Autodesk Fusion 360 part; units mm, degrees
(part 11 of 13)
  line L8940 (111.831, -138.081) -> (111.826, -138.08)
  line L8941 (112.571, -138.625) -> (112.501, -138.633)
  line L8942 (112.241, -138.364) -> (112.216, -138.337)
  line L8943 (111.159, -137.961) -> (111.159, -137.961)
  line L8944 (111.608, -138.003) -> (111.39, -137.964)
  line L8945 (113.035, -138.178) -> (112.933, -138.254)
  line L8946 (112.854, -138.314) -> (112.694, -138.481)
  line L8947 (110.495, -138.178) -> (110.393, -138.254)
  line L8948 (109.961, -138.633) -> (109.897, -138.602)
  line L8949 (111.39, -137.964) -> (111.385, -137.964)
  line L8950 (110.031, -138.625) -> (109.961, -138.633)
  line L8951 (112.626, -138.58) -> (112.571, -138.625)
  line L8952 (112.933, -138.254) -> (112.854, -138.314)
  line L8953 (109.835, -138.513) -> (109.832, -138.508)
  line L8954 (111.312, -137.963) -> (111.159, -137.961)
  line L8955 (112.375, -138.513) -> (112.372, -138.508)
  line L8956 (109.897, -138.602) -> (109.876, -138.577)
  line L8957 (109.812, -138.487) -> (109.701, -138.364)
  line L8958 (112.034, -138.193) -> (112.03, -138.191)
  line L8959 (111.618, -138.006) -> (111.618, -138.006)
  line L8960 (103.048, -123.079) -> (103.053, -123.008)
  line L8961 (103.139, -122.872) -> (103.132, -122.822)
  line L8962 (109.343, -129.567) -> (109.34, -129.559)
  line L8963 (103.096, -122.951) -> (103.146, -122.933)
  line L8964 (109.328, -129.501) -> (109.314, -129.467)
  line L8965 (109.411, -138.147) -> (109.361, -138.097)
  line L8966 (103.144, -117.596) -> (103.151, -117.577)
  line L8967 (109.202, -129.261) -> (109.189, -129.246)
  line L8968 (109.343, -129.575) -> (109.343, -129.567)
  line L8969 (109.346, -129.746) -> (109.346, -129.735)
  line L8970 (102.915, -121.335) -> (103.012, -121.185)
  line L8971 (109.498, -138.197) -> (109.494, -138.193)
  line L8972 (109.346, -129.659) -> (109.346, -129.655)
  line L8973 (103.132, -122.822) -> (103.132, -122.314)
  line L8974 (109.239, -129.314) -> (109.221, -129.282)
  line L8975 (102.906, -122.026) -> (102.849, -121.857)
  line L8976 (109.182, -129.236) -> (109.177, -129.23)
  line L8977 (103.132, -117.697) -> (103.14, -117.647)
  line L8978 (109.348, -129.727) -> (109.346, -129.659)
  line L8979 (103.122, -122.307) -> (102.998, -122.179)
  line L8980 (102.998, -122.179) -> (102.906, -122.026)
  line L8981 (109.344, -129.611) -> (109.343, -129.575)
  line L8982 (109.314, -129.467) -> (109.31, -129.456)
  line L8983 (109.31, -129.456) -> (109.3, -129.421)
  line L8984 (109.328, -129.501) -> (109.328, -129.501)
  line L8985 (109.346, -138.037) -> (109.346, -129.746)
  line L8986 (109.345, -129.623) -> (109.344, -129.611)
  line L8987 (109.298, -129.413) -> (109.288, -129.396)
  line L8988 (109.279, -129.378) -> (109.272, -129.359)
  line L8989 (109.346, -129.655) -> (109.346, -129.627)
  line L8990 (109.337, -129.548) -> (109.333, -129.528)
  line L8991 (109.331, -129.516) -> (109.33, -129.508)
  line L8992 (109.272, -129.359) -> (109.246, -129.324)
  line L8993 (109.288, -129.396) -> (109.279, -129.378)
  line L8994 (109.3, -129.421) -> (109.298, -129.413)
  line L8995 (109.246, -129.324) -> (109.239, -129.314)
  line L8996 (110.7, -138.07) -> (110.7, -138.07)
  line L8997 (109.361, -138.097) -> (109.346, -138.037)
  line L8998 (109.876, -138.577) -> (109.835, -138.513)
  line L8999 (109.346, -129.627) -> (109.345, -129.623)
  line L9000 (109.494, -138.193) -> (109.411, -138.147)
  line L9001 (109.34, -129.559) -> (109.337, -129.548)
  line L9002 (109.34, -129.559) -> (109.34, -129.559)
  line L9003 (109.333, -129.528) -> (109.331, -129.516)
  line L9004 (103.012, -121.185) -> (103.132, -121.068)
  line L9005 (109.33, -129.508) -> (109.328, -129.501)
  line L9006 (103.142, -122.923) -> (103.139, -122.872)
  line L9007 (109.346, -129.735) -> (109.348, -129.727)
  line L9008 (104.249, -109.045) -> (104.184, -109.088)
  line L9009 (109.135, -129.194) -> (103.082, -123.141)
  line L9010 (109.177, -129.23) -> (109.143, -129.202)
  line L9011 (96.4732, -108.552) -> (94.3232, -108.552)
  line L9012 (103.146, -122.933) -> (103.142, -122.923)
  line L9013 (94.3232, -108.552) -> (94.3232, -113.452)
  line L9014 (84.9232, -102.652) -> (94.3232, -102.652)
  line L9015 (103.151, -117.577) -> (103.154, -117.557)
  line L9016 (104.088, -109.107) -> (102.838, -109.107)
  line L9017 (94.3232, -102.652) -> (94.3232, -107.552)
  line L9018 (84.9232, -113.452) -> (84.9232, -102.652)
  line L9019 (102.588, -108.552) -> (101.073, -108.552)
  line L9020 (102.661, -109.034) -> (102.607, -108.953)
  line L9021 (101.073, -108.602) -> (96.4732, -108.602)
  line L9022 (96.4732, -108.602) -> (96.4732, -108.552)
  line L9023 (102.607, -108.953) -> (102.588, -108.857)
  line L9024 (103.082, -123.141) -> (103.048, -123.079)
  line L9025 (109.143, -129.202) -> (109.135, -129.194)
  line L9026 (103.154, -117.557) -> (103.176, -117.511)
  line L9027 (103.132, -121.068) -> (103.132, -117.704)
  line L9028 (109.189, -129.246) -> (109.182, -129.236)
  line L9029 (103.132, -117.704) -> (103.132, -117.697)
  line L9030 (109.221, -129.282) -> (109.221, -129.282)
  line L9031 (103.132, -122.314) -> (103.122, -122.307)
  line L9032 (103.193, -117.463) -> (103.206, -117.447)
  line L9033 (99.2801, -138.842) -> (99.3742, -139.005)
  line L9034 (102.832, -121.679) -> (102.854, -121.502)
  line L9035 (109.221, -129.282) -> (109.217, -129.276)
  line L9036 (109.217, -129.276) -> (109.202, -129.261)
  line L9037 (103.214, -117.429) -> (103.248, -117.391)
  line L9038 (102.742, -109.088) -> (102.661, -109.034)
  line L9039 (103.14, -117.647) -> (103.144, -117.596)
  line L9040 (103.206, -117.447) -> (103.214, -117.429)
  line L9041 (102.849, -121.857) -> (102.832, -121.679)
  line L9042 (103.053, -123.008) -> (103.096, -122.951)
  line L9043 (104.184, -109.088) -> (104.088, -109.107)
  line L9044 (99.1542, -138.702) -> (99.2801, -138.842)
  line L9045 (104.96, -109.045) -> (104.249, -109.045)
  line L9046 (102.838, -109.107) -> (102.742, -109.088)
  line L9047 (105.951, -114.677) -> (105.951, -110.037)
  line L9048 (103.176, -117.511) -> (103.193, -117.463)
  line L9049 (103.248, -117.391) -> (103.278, -117.35)
  line L9050 (102.854, -121.502) -> (102.915, -121.335)
  line L9051 (103.278, -117.35) -> (105.951, -114.677)
  line L9052 (98.8301, -138.515) -> (99.002, -138.591)
  line L9053 (105.951, -110.037) -> (104.96, -109.045)
  line L9054 (102.588, -108.857) -> (102.588, -108.552)
  line L9055 (101.073, -108.552) -> (101.073, -108.602)
  line L9056 (113.064, -138.842) -> (113.19, -138.702)
  line L9057 (111.854, -138.702) -> (111.98, -138.842)
  line L9058 (113.886, -140.266) -> (113.698, -140.266)
  line L9059 (112.97, -139.005) -> (113.064, -138.842)
  line L9060 (114.242, -140.15) -> (114.07, -140.227)
  line L9061 (97.8239, -139.9) -> (97.7298, -139.737)
  line L9062 (98.6461, -140.266) -> (98.4579, -140.266)
  line L9063 (99.002, -138.591) -> (99.1542, -138.702)
  line L9064 (114.394, -138.702) -> (114.52, -138.842)
  line L9065 (98.2739, -140.227) -> (98.102, -140.15)
  line L9066 (114.242, -138.591) -> (114.394, -138.702)
  line L9067 (111.98, -138.842) -> (112.074, -139.005)
  line L9068 (98.2739, -138.515) -> (98.4579, -138.476)
  line L9069 (97.6717, -139.558) -> (97.652, -139.371)
  line L9070 (114.672, -139.183) -> (114.692, -139.371)
  line L9071 (114.614, -139.737) -> (114.52, -139.9)
  line L9072 (97.7298, -139.005) -> (97.8239, -138.842)
  line L9073 (114.614, -139.005) -> (114.672, -139.183)
  line L9074 (98.4579, -138.476) -> (98.6461, -138.476)
  line L9075 (98.102, -138.591) -> (98.2739, -138.515)
  line L9076 (113.514, -138.515) -> (113.698, -138.476)
  line L9077 (97.9498, -138.702) -> (98.102, -138.591)
  line L9078 (114.07, -138.515) -> (114.242, -138.591)
  line L9079 (99.2801, -139.9) -> (99.1542, -140.039)
  line L9080 (97.7298, -139.737) -> (97.6717, -139.558)
  line L9081 (98.8301, -140.227) -> (98.6461, -140.266)
  line L9082 (114.52, -138.842) -> (114.614, -139.005)
  line L9083 (99.452, -139.371) -> (99.4323, -139.558)
  line L9084 (97.8239, -138.842) -> (97.9498, -138.702)
  line L9085 (112.97, -139.737) -> (112.912, -139.558)
  line L9086 (94.3232, -113.452) -> (84.9232, -113.452)
  line L9087 (113.342, -140.15) -> (113.19, -140.039)
  line L9088 (112.132, -139.558) -> (112.074, -139.737)
  line L9089 (97.6717, -139.183) -> (97.7298, -139.005)
  line L9090 (114.692, -139.371) -> (114.672, -139.558)
  line L9091 (113.064, -139.9) -> (112.97, -139.737)
  line L9092 (97.9498, -140.039) -> (97.8239, -139.9)
  line L9093 (99.1542, -140.039) -> (99.002, -140.15)
  line L9094 (99.3742, -139.737) -> (99.2801, -139.9)
  line L9095 (99.4323, -139.183) -> (99.452, -139.371)
  line L9096 (99.4323, -139.558) -> (99.3742, -139.737)
  line L9097 (99.002, -140.15) -> (98.8301, -140.227)
  line L9098 (112.912, -139.183) -> (112.97, -139.005)
  line L9099 (98.4579, -140.266) -> (98.2739, -140.227)
  line L9100 (98.102, -140.15) -> (97.9498, -140.039)
  line L9101 (99.3742, -139.005) -> (99.4323, -139.183)
  line L9102 (98.6461, -138.476) -> (98.8301, -138.515)
  line L9103 (97.652, -139.371) -> (97.6717, -139.183)
  line L9104 (110.802, -138.591) -> (110.974, -138.515)
  line L9105 (114.07, -140.227) -> (113.886, -140.266)
  line L9106 (112.132, -139.183) -> (112.152, -139.371)
  line L9107 (113.19, -138.702) -> (113.342, -138.591)
  line L9108 (113.698, -138.476) -> (113.886, -138.476)
  line L9109 (111.53, -138.515) -> (111.702, -138.591)
  line L9110 (112.074, -139.005) -> (112.132, -139.183)
  line L9111 (102.994, -115.901) -> (103.105, -115.958)
  line L9112 (110.372, -139.183) -> (110.43, -139.005)
  line L9113 (110.43, -139.737) -> (110.372, -139.558)
  line L9114 (103.105, -116.605) -> (102.994, -116.662)
  line L9115 (111.346, -138.476) -> (111.53, -138.515)
  line L9116 (111.702, -140.15) -> (111.53, -140.227)
  line L9117 (103.25, -116.158) -> (103.27, -116.281)
  line L9118 (103.27, -116.281) -> (103.25, -116.405)
  line L9119 (103.25, -116.405) -> (103.194, -116.516)
  line L9120 (110.802, -140.15) -> (110.65, -140.039)
  line L9121 (111.702, -138.591) -> (111.854, -138.702)
  line L9122 (110.43, -139.005) -> (110.524, -138.842)
  line L9123 (112.074, -139.737) -> (111.98, -139.9)
  line L9124 (102.87, -116.681) -> (102.746, -116.662)
  line L9125 (112.152, -139.371) -> (112.132, -139.558)
  line L9126 (113.342, -138.591) -> (113.514, -138.515)
  line L9127 (114.672, -139.558) -> (114.614, -139.737)
  line L9128 (103.105, -115.958) -> (103.194, -116.046)
  line L9129 (103.194, -116.046) -> (103.25, -116.158)
  line L9130 (103.194, -116.516) -> (103.105, -116.605)
  line L9131 (111.854, -140.039) -> (111.702, -140.15)
  line L9132 (111.158, -140.266) -> (110.974, -140.227)
  line L9133 (111.98, -139.9) -> (111.854, -140.039)
  line L9134 (110.524, -139.9) -> (110.43, -139.737)
  line L9135 (112.892, -139.371) -> (112.912, -139.183)
  line L9136 (114.52, -139.9) -> (114.394, -140.039)
  line L9137 (113.19, -140.039) -> (113.064, -139.9)
  line L9138 (102.994, -116.662) -> (102.87, -116.681)
  line L9139 (110.352, -139.371) -> (110.372, -139.183)
  line L9140 (110.974, -138.515) -> (111.158, -138.476)
  line L9141 (113.886, -138.476) -> (114.07, -138.515)
  line L9142 (113.514, -140.227) -> (113.342, -140.15)
  line L9143 (110.524, -138.842) -> (110.65, -138.702)
  line L9144 (112.912, -139.558) -> (112.892, -139.371)
  line L9145 (111.53, -140.227) -> (111.346, -140.266)
  line L9146 (113.698, -140.266) -> (113.514, -140.227)
  line L9147 (110.65, -138.702) -> (110.802, -138.591)
  line L9148 (110.372, -139.558) -> (110.352, -139.371)
  line L9149 (110.65, -140.039) -> (110.524, -139.9)
  line L9150 (114.394, -140.039) -> (114.242, -140.15)
  line L9151 (111.346, -140.266) -> (111.158, -140.266)
  line L9152 (102.553, -123.685) -> (102.129, -123.26)
  line L9153 (102.342, -123.12) -> (102.73, -123.508)
  line L9154 (108.818, -129.602) -> (108.822, -129.607)
  line L9155 (108.837, -129.667) -> (108.837, -138.482)
  line L9156 (107.984, -139.9) -> (107.89, -139.737)
  line L9157 (102.73, -123.508) -> (108.8, -129.579)
  line L9158 (109.162, -140.15) -> (108.99, -140.227)
  line L9159 (109.44, -139.9) -> (109.314, -140.039)
  line L9160 (102.517, -116.458) -> (102.49, -116.405)
  line L9161 (102.693, -116.635) -> (102.342, -116.986)
  line L9162 (111.158, -138.476) -> (111.346, -138.476)
  line L9163 (109.592, -139.183) -> (109.612, -139.371)
  line L9164 (108.262, -140.15) -> (108.11, -140.039)
  line L9165 (108.8, -129.579) -> (108.814, -129.596)
  line L9166 (102.097, -116.899) -> (102.114, -116.873)
  line L9167 (102.47, -116.281) -> (102.49, -116.158)
  line L9168 (108.99, -138.515) -> (109.162, -138.591)
  line L9169 (108.618, -140.266) -> (108.434, -140.227)
  line L9170 (108.99, -140.227) -> (108.806, -140.266)
  line L9171 (110.974, -140.227) -> (110.802, -140.15)
  line L9172 (109.314, -138.702) -> (109.44, -138.842)
  line L9173 (108.828, -129.637) -> (108.837, -129.667)
  line L9174 (109.162, -138.591) -> (109.314, -138.702)
  line L9175 (108.434, -138.515) -> (108.587, -138.482)
  line L9176 (102.73, -123.508) -> (102.73, -123.508)
  line L9177 (107.812, -139.371) -> (107.832, -139.183)
  line L9178 (109.612, -139.371) -> (109.592, -139.558)
  line L9179 (108.434, -140.227) -> (108.262, -140.15)
  line L9180 (108.837, -138.482) -> (108.99, -138.515)
  line L9181 (109.44, -138.842) -> (109.534, -139.005)
  line L9182 (102.49, -116.405) -> (102.47, -116.281)
  line L9183 (108.11, -138.702) -> (108.262, -138.591)
  line L9184 (109.592, -139.558) -> (109.534, -139.737)
  line L9185 (109.534, -139.737) -> (109.44, -139.9)
  line L9186 (102.342, -116.986) -> (102.342, -123.12)
  line L9187 (102.129, -123.26) -> (102.115, -123.243)
  line L9188 (108.262, -138.591) -> (108.434, -138.515)
  line L9189 (108.817, -129.599) -> (108.818, -129.602)
  line L9190 (109.534, -139.005) -> (109.592, -139.183)
  line L9191 (102.111, -123.237) -> (102.107, -123.232)
  line L9192 (108.822, -129.607) -> (108.828, -129.637)
  line L9193 (109.314, -140.039) -> (109.162, -140.15)
  line L9194 (108.814, -129.596) -> (108.817, -129.599)
  line L9195 (102.553, -123.685) -> (102.553, -123.685)
  line L9196 (102.746, -116.662) -> (102.693, -116.635)
  line L9197 (102.107, -123.232) -> (102.101, -123.202)
  line L9198 (108.806, -140.266) -> (108.618, -140.266)
  line L9199 (108.11, -140.039) -> (107.984, -139.9)
  line L9200 (105.894, -138.515) -> (106.078, -138.476)
  line L9201 (106.622, -140.15) -> (106.45, -140.227)
  line L9202 (106.994, -139.737) -> (106.9, -139.9)
  line L9203 (102.87, -115.881) -> (102.994, -115.901)
  line L9204 (105.444, -138.842) -> (105.57, -138.702)
  line L9205 (102.092, -116.934) -> (102.095, -116.912)
  line L9206 (106.622, -138.591) -> (106.774, -138.702)
  line L9207 (105.57, -138.702) -> (105.722, -138.591)
  line L9208 (105.722, -138.591) -> (105.894, -138.515)
  line L9209 (102.115, -123.243) -> (102.112, -123.24)
  line L9210 (102.546, -116.046) -> (102.635, -115.958)
  line L9211 (102.746, -115.901) -> (102.87, -115.881)
  line L9212 (107.832, -139.183) -> (107.89, -139.005)
  line L9213 (106.774, -138.702) -> (106.9, -138.842)
  line L9214 (102.114, -116.873) -> (102.129, -116.846)
  line L9215 (108.587, -138.482) -> (108.587, -129.719)
  line L9216 (105.292, -139.183) -> (105.35, -139.005)
  line L9217 (107.89, -139.005) -> (107.984, -138.842)
  line L9218 (102.129, -116.846) -> (102.517, -116.458)
  line L9219 (102.095, -116.912) -> (102.095, -116.908)
  line L9220 (106.994, -139.005) -> (107.052, -139.183)
  line L9221 (105.292, -139.558) -> (105.272, -139.371)
  line L9222 (105.57, -140.039) -> (105.444, -139.9)
  line L9223 (102.112, -123.24) -> (102.111, -123.237)
  line L9224 (102.095, -116.908) -> (102.096, -116.905)
  line L9225 (107.984, -138.842) -> (108.11, -138.702)
  line L9226 (106.774, -140.039) -> (106.622, -140.15)
  line L9227 (107.072, -139.371) -> (107.052, -139.558)
  line L9228 (105.722, -140.15) -> (105.57, -140.039)
  line L9229 (107.052, -139.558) -> (106.994, -139.737)
  line L9230 (102.635, -115.958) -> (102.746, -115.901)
  line L9231 (105.894, -140.227) -> (105.722, -140.15)
  line L9232 (105.35, -139.737) -> (105.292, -139.558)
  line L9233 (107.052, -139.183) -> (107.072, -139.371)
  line L9234 (105.444, -139.9) -> (105.35, -139.737)
  line L9235 (106.45, -138.515) -> (106.622, -138.591)
  line L9236 (102.101, -123.202) -> (102.092, -123.172)
  line L9237 (107.89, -139.737) -> (107.832, -139.558)
  line L9238 (106.45, -140.227) -> (106.266, -140.266)
  line L9239 (108.587, -129.719) -> (102.553, -123.685)
  line L9240 (102.49, -116.158) -> (102.546, -116.046)
  line L9241 (107.832, -139.558) -> (107.812, -139.371)
  line L9242 (106.078, -140.266) -> (105.894, -140.227)
  line L9243 (105.272, -139.371) -> (105.292, -139.183)
  line L9244 (102.092, -123.172) -> (102.092, -116.934)
  line L9245 (102.096, -116.905) -> (102.097, -116.899)
  line L9246 (106.9, -138.842) -> (106.994, -139.005)
  line L9247 (105.35, -139.005) -> (105.444, -138.842)
  line L9248 (100.248, -122.697) -> (100.252, -122.7)
  line L9249 (100.864, -122.984) -> (101.092, -123.004)
  line L9250 (99.891, -122.256) -> (99.9362, -122.308)
  line L9251 (101.585, -123.228) -> (101.586, -123.272)
  line L9252 (101.635, -123.432) -> (101.641, -123.443)
  line L9253 (101.596, -123.311) -> (101.599, -123.331)
  line L9254 (101.641, -123.443) -> (101.65, -123.461)
  line L9255 (101.496, -122.958) -> (101.555, -122.998)
  line L9256 (101.092, -123.004) -> (101.32, -122.984)
  line L9257 (106.266, -140.266) -> (106.078, -140.266)
  line L9258 (100.44, -122.83) -> (100.44, -122.83)
  line L9259 (99.9522, -122.342) -> (99.9545, -122.347)
  line L9260 (101.555, -122.998) -> (101.583, -123.063)
  line L9261 (106.9, -139.9) -> (106.774, -140.039)
  line L9262 (100.6, -122.905) -> (100.643, -122.925)
  line L9263 (101.584, -123.093) -> (101.583, -123.104)
  line L9264 (106.266, -138.476) -> (106.45, -138.515)
  line L9265 (99.9576, -122.352) -> (100.074, -122.518)
  line L9266 (100.648, -122.926) -> (100.648, -122.926)
  line L9267 (100.643, -122.925) -> (100.648, -122.926)
  line L9268 (101.425, -122.956) -> (101.496, -122.958)
  line L9269 (101.583, -123.063) -> (101.584, -123.078)
  line L9270 (100.252, -122.7) -> (100.252, -122.7)
  line L9271 (100.435, -122.828) -> (100.44, -122.83)
  line L9272 (101.619, -123.383) -> (101.631, -123.426)
  line L9273 (101.584, -123.078) -> (101.584, -123.093)
  line L9274 (99.9522, -122.342) -> (99.9522, -122.342)
  line L9275 (101.584, -123.184) -> (101.584, -123.212)
  line L9276 (101.581, -123.112) -> (101.582, -123.12)
  line L9277 (101.601, -123.338) -> (101.601, -123.338)
  line L9278 (101.635, -123.432) -> (101.635, -123.432)
  line L9279 (101.586, -123.272) -> (101.592, -123.291)
  line L9280 (100.31, -122.741) -> (100.435, -122.828)
  line L9281 (99.9362, -122.308) -> (99.9522, -122.342)
  line L9282 (100.074, -122.518) -> (100.086, -122.535)
  line L9283 (99.9545, -122.347) -> (99.9576, -122.352)
  line L9284 (100.859, -122.983) -> (100.859, -122.983)
  line L9285 (106.078, -138.476) -> (106.266, -138.476)
  line L9286 (100.859, -122.983) -> (100.864, -122.984)
  line L9287 (100.44, -122.83) -> (100.6, -122.905)
  line L9288 (101.32, -122.984) -> (101.425, -122.956)
  line L9289 (100.252, -122.7) -> (100.31, -122.741)
  line L9290 (100.648, -122.926) -> (100.859, -122.983)
  line L9291 (101.631, -123.426) -> (101.635, -123.432)
  line L9292 (101.583, -123.104) -> (101.581, -123.112)
  line L9293 (101.584, -123.216) -> (101.584, -123.216)
  line L9294 (101.657, -123.48) -> (101.662, -123.486)
  line L9295 (100.086, -122.535) -> (100.248, -122.697)
  line L9296 (102.137, -123.988) -> (108.042, -129.892)
  line L9297 (107.295, -138.513) -> (107.292, -138.508)
  line L9298 (107.614, -138.481) -> (107.546, -138.58)
  line L9299 (107.546, -138.58) -> (107.491, -138.625)
  line L9300 (101.601, -123.338) -> (101.615, -123.372)
  line L9301 (101.74, -123.593) -> (101.752, -123.609)
  line L9302 (108.058, -138.104) -> (108.011, -138.148)
  line L9303 (101.712, -123.563) -> (101.727, -123.578)
  line L9304 (107.357, -138.602) -> (107.336, -138.577)
  line L9305 (101.583, -123.18) -> (101.584, -123.184)
  line L9306 (107.959, -138.175) -> (107.955, -138.178)
  line L9307 (101.599, -123.331) -> (101.601, -123.338)
  line L9308 (101.615, -123.372) -> (101.619, -123.383)
  line L9309 (101.584, -123.216) -> (101.584, -123.216)
  line L9310 (101.683, -123.515) -> (101.69, -123.525)
  line L9311 (101.662, -123.486) -> (101.683, -123.515)
  line L9312 (107.963, -138.172) -> (107.959, -138.175)
  line L9313 (108.011, -138.148) -> (107.963, -138.172)
  line L9314 (108.078, -138.036) -> (108.058, -138.104)
  line L9315 (107.272, -138.487) -> (107.161, -138.364)
  line L9316 (108.076, -129.955) -> (108.078, -129.982)
  line L9317 (101.758, -123.614) -> (101.786, -123.637)
  line L9318 (107.491, -138.625) -> (107.421, -138.633)
  line L9319 (101.65, -123.461) -> (101.657, -123.48)
  line L9320 (107.877, -138.236) -> (107.774, -138.314)
  line L9321 (107.292, -138.508) -> (107.272, -138.487)
  line L9322 (107.774, -138.314) -> (107.614, -138.481)
  line L9323 (101.69, -123.525) -> (101.712, -123.563)
  line L9324 (101.584, -123.216) -> (101.585, -123.228)
  line L9325 (101.786, -123.637) -> (101.794, -123.645)
  line L9326 (101.582, -123.12) -> (101.583, -123.18)
  line L9327 (101.584, -123.212) -> (101.584, -123.216)
  line L9328 (101.592, -123.291) -> (101.596, -123.311)
  line L9329 (101.794, -123.645) -> (102.137, -123.988)
  line L9330 (107.421, -138.633) -> (107.357, -138.602)
  line L9331 (101.727, -123.578) -> (101.74, -123.593)
  line L9332 (101.662, -123.486) -> (101.662, -123.486)
  line L9333 (101.582, -123.12) -> (101.582, -123.12)
  line L9334 (107.955, -138.178) -> (107.955, -138.178)
  line L9335 (143.647, -107.958) -> (143.617, -107.965)
  line L9336 (146.657, -97.0052) -> (146.58, -97.0204)
  line L9337 (146.58, -97.0204) -> (146.18, -97.0204)
  line L9338 (145.842, -97.9436) -> (145.841, -97.9461)
  line L9339 (145.98, -96.8204) -> (145.98, -96.6704)
  line L9340 (144.928, -106.657) -> (144.926, -106.66)
  line L9341 (141.756, -124.03) -> (143.626, -122.159)
  line L9342 (144.925, -106.666) -> (144.909, -106.692)
  line L9343 (143.102, -107.973) -> (142.568, -108.508)
  line L9344 (146.104, -97.0052) -> (146.039, -96.9618)
  line L9345 (145.98, -96.6704) -> (145.845, -96.6704)
  line L9346 (145.995, -96.8969) -> (145.98, -96.8204)
  line L9347 (145.845, -96.6704) -> (145.845, -97.917)
  line L9348 (146.104, -96.0856) -> (146.18, -96.0704)
  line L9349 (146.722, -96.9618) -> (146.657, -97.0052)
  line L9350 (146.18, -97.0204) -> (146.104, -97.0052)
  line L9351 (122.753, -122.378) -> (122.752, -122.381)
  line L9352 (122.734, -122.413) -> (122.72, -122.44)
  line L9353 (143.658, -107.95) -> (143.655, -107.954)
  line L9354 (107.185, -117.298) -> (107.296, -117.355)
  line L9355 (143.588, -107.973) -> (143.102, -107.973)
  line L9356 (107.689, -118.134) -> (107.692, -118.137)
  line L9357 (146.765, -96.1939) -> (146.78, -96.2704)
  line L9358 (145.841, -97.9461) -> (145.84, -97.9525)
  line L9359 (146.765, -96.8969) -> (146.722, -96.9618)
  line L9360 (143.655, -107.954) -> (143.653, -107.954)
  line L9361 (145.845, -97.917) -> (145.842, -97.939)
  line L9362 (144.93, -98.8832) -> (144.93, -106.631)
  line L9363 (146.039, -96.9618) -> (145.995, -96.8969)
  line L9364 (144.93, -106.631) -> (144.927, -106.653)
  line L9365 (145.842, -97.939) -> (145.842, -97.9436)
  line L9366 (143.617, -107.965) -> (143.588, -107.973)
  line L9367 (144.927, -106.653) -> (144.928, -106.657)
  line L9368 (145.823, -97.9784) -> (145.808, -98.0054)
  line L9369 (107.675, -118.116) -> (107.689, -118.134)
  line L9370 (107.693, -118.139) -> (107.697, -118.145)
  line L9371 (145.84, -97.9525) -> (145.823, -97.9784)
  line L9372 (144.894, -106.719) -> (143.676, -107.937)
  line L9373 (145.808, -98.0054) -> (144.93, -98.8832)
  line L9374 (146.78, -96.2704) -> (146.78, -96.8204)
  line L9375 (107.692, -118.137) -> (107.693, -118.139)
  line L9376 (146.58, -96.0704) -> (146.657, -96.0856)
  line L9377 (144.909, -106.692) -> (144.894, -106.719)
  line L9378 (143.676, -107.937) -> (143.658, -107.95)
  line L9379 (108.038, -123.102) -> (108.967, -124.03)
  line L9380 (144.926, -106.66) -> (144.925, -106.666)
  line L9381 (146.657, -96.0856) -> (146.722, -96.129)
  line L9382 (143.653, -107.954) -> (143.647, -107.958)
  line L9383 (122.756, -122.352) -> (122.753, -122.374)
  line L9384 (142.546, -112.787) -> (142.532, -112.814)
  line L9385 (133.148, -113.968) -> (130.702, -116.413)
  line L9386 (130.614, -116.45) -> (123.809, -116.45)
  line L9387 (122.753, -122.374) -> (122.753, -122.378)
  line L9388 (141.414, -113.931) -> (141.396, -113.945)
  line L9389 (121.924, -123.205) -> (121.895, -123.213)
  line L9390 (114.261, -122.337) -> (114.122, -122.419)
  line L9391 (113.953, -122.474) -> (113.775, -122.49)
  line L9392 (115.094, -123.169) -> (114.261, -122.337)
  line L9393 (122.751, -122.387) -> (122.734, -122.413)
  line L9394 (142.568, -112.725) -> (142.565, -112.747)
  line L9395 (114.122, -122.419) -> (113.953, -122.474)
  line L9396 (122.756, -117.503) -> (122.756, -122.352)
  line L9397 (142.565, -112.747) -> (142.565, -112.752)
  line L9398 (121.983, -123.177) -> (121.965, -123.19)
  line L9399 (141.385, -113.953) -> (141.355, -113.959)
  line L9400 (130.682, -116.43) -> (130.679, -116.431)
  line L9401 (142.565, -112.752) -> (142.564, -112.754)
  line L9402 (142.564, -112.754) -> (142.563, -112.761)
  line L9403 (141.355, -113.959) -> (141.326, -113.968)
  line L9404 (122.752, -122.381) -> (122.751, -122.387)
  line L9405 (130.685, -116.427) -> (130.682, -116.43)
  line L9406 (130.679, -116.431) -> (130.674, -116.435)
  line L9407 (142.563, -112.761) -> (142.546, -112.787)
  line L9408 (130.674, -116.435) -> (130.644, -116.441)
  line L9409 (141.39, -113.949) -> (141.385, -113.953)
  line L9410 (123.809, -116.45) -> (122.756, -117.503)
  line L9411 (115.162, -123.209) -> (115.153, -123.208)
  line L9412 (121.965, -123.19) -> (121.962, -123.194)
  line L9413 (115.153, -123.208) -> (115.146, -123.203)
  line L9414 (115.137, -123.202) -> (115.118, -123.185)
  line L9415 (115.189, -123.213) -> (115.163, -123.21)
  line L9416 (142.532, -112.814) -> (141.414, -113.931)
  line L9417 (113.431, -122.405) -> (113.282, -122.307)
  line L9418 (115.118, -123.185) -> (115.101, -123.176)
  line L9419 (121.895, -123.213) -> (115.189, -123.213)
  line L9420 (115.095, -123.171) -> (115.094, -123.17)
  line L9421 (130.644, -116.441) -> (130.614, -116.45)
  line L9422 (141.326, -113.968) -> (133.148, -113.968)
  line L9423 (113.775, -122.49) -> (113.598, -122.467)
  line L9424 (115.094, -123.17) -> (115.094, -123.169)
  line L9425 (141.396, -113.945) -> (141.393, -113.948)
  line L9426 (122.72, -122.44) -> (121.983, -123.177)
  line L9427 (130.702, -116.413) -> (130.685, -116.427)
  line L9428 (115.101, -123.176) -> (115.095, -123.171)
  line L9429 (141.393, -113.948) -> (141.39, -113.949)
  line L9430 (142.568, -108.508) -> (142.568, -112.725)
  line L9431 (123.693, -116.219) -> (123.698, -116.215)
  line L9432 (113.62, -120.909) -> (113.798, -120.891)
  line L9433 (113.158, -122.179) -> (113.066, -122.026)
  line L9434 (123.698, -116.215) -> (123.728, -116.208)
  line L9435 (113.975, -120.912) -> (114.143, -120.972)
  line L9436 (123.728, -116.208) -> (123.757, -116.2)
  line L9437 (113.798, -120.891) -> (113.975, -120.912)
  line L9438 (143.536, -107.723) -> (144.68, -106.579)
  line L9439 (123.757, -116.2) -> (130.562, -116.2)
  line L9440 (113.014, -121.502) -> (113.075, -121.335)
  line L9441 (123.669, -116.236) -> (123.687, -116.223)
  line L9442 (113.009, -121.857) -> (112.992, -121.679)
  line L9443 (114.143, -120.972) -> (114.293, -121.067)
  line L9444 (114.513, -121.345) -> (114.572, -121.513)
  line L9445 (115.146, -123.203) -> (115.137, -123.202)
  line L9446 (114.293, -121.067) -> (114.419, -121.194)
  line L9447 (114.592, -121.691) -> (114.592, -121.713)
  line L9448 (113.451, -120.967) -> (113.62, -120.909)
  line L9449 (114.436, -122.158) -> (115.242, -122.963)
  line L9450 (122.511, -117.415) -> (122.528, -117.39)
  line L9451 (122.509, -117.424) -> (122.51, -117.422)
  line L9452 (122.528, -117.39) -> (122.543, -117.363)
  line L9453 (114.419, -121.194) -> (114.513, -121.345)
  line L9454 (113.598, -122.467) -> (113.431, -122.405)
  line L9455 (114.572, -121.513) -> (114.592, -121.691)
  line L9456 (121.959, -123.194) -> (121.954, -123.198)
  line L9457 (113.066, -122.026) -> (113.009, -121.857)
  line L9458 (115.163, -123.21) -> (115.162, -123.21)
  line L9459 (113.075, -121.335) -> (113.172, -121.185)
  line L9460 (121.843, -122.963) -> (122.506, -122.3)
  line L9461 (122.51, -117.422) -> (122.511, -117.415)
  line L9462 (114.567, -121.89) -> (114.504, -122.056)
  line L9463 (123.69, -116.22) -> (123.693, -116.219)
  line L9464 (121.962, -123.194) -> (121.959, -123.194)
  line L9465 (115.162, -123.21) -> (115.162, -123.209)
  line L9466 (113.299, -121.06) -> (113.451, -120.967)
  line L9467 (114.592, -121.713) -> (114.567, -121.89)
  line L9468 (122.543, -117.363) -> (123.669, -116.236)
  line L9469 (123.687, -116.223) -> (123.69, -116.22)
  line L9470 (112.992, -121.679) -> (113.014, -121.502)
  line L9471 (113.172, -121.185) -> (113.299, -121.06)
  line L9472 (122.509, -117.429) -> (122.509, -117.424)
  line L9473 (121.954, -123.198) -> (121.924, -123.205)
  line L9474 (122.506, -117.451) -> (122.509, -117.429)
  line L9475 (113.282, -122.307) -> (113.158, -122.179)
  line L9476 (122.506, -122.3) -> (122.506, -117.451)
  line L9477 (115.242, -122.963) -> (121.843, -122.963)
  line L9478 (114.504, -122.056) -> (114.436, -122.158)
  line L9479 (133.025, -113.741) -> (133.028, -113.738)
  line L9480 (133.008, -113.754) -> (133.025, -113.741)
  line L9481 (142.318, -112.673) -> (142.318, -108.456)
  line L9482 (142.98, -107.747) -> (142.983, -107.743)
  line L9483 (145.056, -97.0052) -> (144.979, -97.0204)
  line L9484 (145.179, -96.4204) -> (145.98, -96.4204)
  line L9485 (145.056, -96.0856) -> (145.12, -96.129)
  line L9486 (144.68, -98.8314) -> (144.684, -98.8094)
  line L9487 (142.321, -108.429) -> (142.322, -108.427)
  line L9488 (106.799, -121.194) -> (106.893, -121.345)
  line L9489 (142.318, -108.456) -> (142.321, -108.434)
  line L9490 (133.031, -113.737) -> (133.036, -113.733)
  line L9491 (143.051, -107.723) -> (143.536, -107.723)
  line L9492 (144.502, -96.0856) -> (144.579, -96.0704)
  line L9493 (133.028, -113.738) -> (133.031, -113.737)
  line L9494 (142.991, -107.739) -> (143.021, -107.732)
  line L9495 (106.355, -120.912) -> (106.523, -120.972)
  line L9496 (145.164, -96.1939) -> (145.179, -96.2704)
  line L9497 (145.179, -96.6704) -> (145.179, -96.8204)
  line L9498 (144.394, -96.8969) -> (144.379, -96.8204)
  line L9499 (144.68, -106.579) -> (144.68, -98.8314)
  line L9500 (144.686, -98.7959) -> (144.702, -98.77)
  line L9501 (144.683, -98.8048) -> (144.685, -98.8023)
  line L9502 (133.036, -113.733) -> (133.066, -113.726)
  line L9503 (141.274, -113.718) -> (142.318, -112.673)
  line L9504 (142.983, -107.743) -> (142.986, -107.742)
  line L9505 (142.355, -108.367) -> (142.962, -107.76)
  line L9506 (143.021, -107.732) -> (143.051, -107.723)
  line L9507 (142.962, -107.76) -> (142.98, -107.747)
  line L9508 (133.066, -113.726) -> (133.096, -113.718)
  line L9509 (142.321, -108.434) -> (142.321, -108.429)
  line L9510 (144.979, -96.0704) -> (145.056, -96.0856)
  line L9511 (142.322, -108.427) -> (142.323, -108.42)
  line L9512 (144.979, -97.0204) -> (144.579, -97.0204)
  line L9513 (133.096, -113.718) -> (141.274, -113.718)
  line L9514 (144.684, -98.8094) -> (144.683, -98.8048)
  line L9515 (106.523, -120.972) -> (106.673, -121.067)
  line L9516 (130.562, -116.2) -> (133.008, -113.754)
  line L9517 (106.673, -121.067) -> (106.799, -121.194)
  line L9518 (142.986, -107.742) -> (142.991, -107.739)
  line L9519 (145.12, -96.9618) -> (145.056, -97.0052)
  line L9520 (142.34, -108.394) -> (142.355, -108.367)
  line L9521 (144.685, -98.8023) -> (144.686, -98.7959)
  line L9522 (142.323, -108.42) -> (142.34, -108.394)
  line L9523 (145.12, -96.129) -> (145.164, -96.1939)
  line L9524 (145.98, -96.4204) -> (145.98, -96.2704)
  line L9525 (144.394, -96.1939) -> (144.438, -96.129)
  line L9526 (106.893, -121.345) -> (106.952, -121.513)
  line L9527 (124.093, -113.545) -> (124.065, -113.527)
  line L9528 (105.389, -121.857) -> (105.372, -121.679)
  line L9529 (106.947, -121.89) -> (106.884, -122.056)
  line L9530 (106.502, -122.419) -> (106.333, -122.474)
  line L9531 (128.323, -112.685) -> (128.302, -112.711)
  line L9532 (123.774, -113.354) -> (123.673, -113.338)
  line L9533 (144.579, -96.0704) -> (144.979, -96.0704)
  line L9534 (127.497, -113.527) -> (127.468, -113.545)
  line L9535 (106.884, -122.056) -> (106.785, -122.205)
  line L9536 (127.431, -113.568) -> (127.421, -113.574)
  line L9537 (105.811, -122.405) -> (105.662, -122.307)
  line L9538 (144.717, -98.743) -> (145.595, -97.8652)
  line L9539 (106.178, -120.891) -> (106.355, -120.912)
  line L9540 (127.356, -113.586) -> (124.206, -113.586)
  line L9541 (98.7347, -120.912) -> (98.9027, -120.972)
  line L9542 (106.785, -122.205) -> (106.656, -122.328)
  line L9543 (144.379, -96.8204) -> (144.379, -96.2704)
  line L9544 (105.552, -121.185) -> (105.679, -121.06)
  line L9545 (105.662, -122.307) -> (105.538, -122.179)
  line L9546 (105.679, -121.06) -> (105.831, -120.967)
  line L9547 (144.379, -96.2704) -> (144.394, -96.1939)
  line L9548 (144.438, -96.129) -> (144.502, -96.0856)
  line L9549 (144.579, -97.0204) -> (144.502, -97.0052)
  line L9550 (145.595, -96.6704) -> (145.179, -96.6704)
  line L9551 (105.372, -121.679) -> (105.394, -121.502)
  line L9552 (106, -120.909) -> (106.178, -120.891)
  line L9553 (106.656, -122.328) -> (106.502, -122.419)
  line L9554 (144.438, -96.9618) -> (144.394, -96.8969)
  line L9555 (145.179, -96.2704) -> (145.179, -96.4204)
  line L9556 (105.394, -121.502) -> (105.455, -121.335)
  line L9557 (105.978, -122.467) -> (105.811, -122.405)
  line L9558 (124.206, -113.586) -> (124.173, -113.578)
  line L9559 (105.831, -120.967) -> (106, -120.909)
  line L9560 (124.119, -113.566) -> (124.093, -113.545)
  line L9561 (106.952, -121.513) -> (106.972, -121.691)
  line L9562 (105.455, -121.335) -> (105.552, -121.185)
  line L9563 (144.702, -98.77) -> (144.717, -98.743)
  line L9564 (145.179, -96.8204) -> (145.164, -96.8969)
  line L9565 (144.502, -97.0052) -> (144.438, -96.9618)
  line L9566 (145.164, -96.8969) -> (145.12, -96.9618)
  line L9567 (105.446, -122.026) -> (105.389, -121.857)
  line L9568 (106.155, -122.49) -> (105.978, -122.467)
  line L9569 (106.972, -121.713) -> (106.947, -121.89)
  line L9570 (145.595, -97.8652) -> (145.595, -96.6704)
  line L9571 (106.333, -122.474) -> (106.155, -122.49)
  line L9572 (106.972, -121.691) -> (106.972, -121.713)
  line L9573 (105.538, -122.179) -> (105.446, -122.026)
  line L9574 (127.442, -113.566) -> (127.431, -113.568)
  line L9575 (128.332, -112.664) -> (128.326, -112.674)
  line L9576 (149.446, -115.083) -> (149.43, -115.109)
  line L9577 (128.343, -111.208) -> (128.343, -112.599)
  line L9578 (149.449, -115.075) -> (149.447, -115.077)
  line L9579 (135.93, -110.817) -> (128.734, -110.817)
  line L9580 (149.433, -104.456) -> (149.436, -104.461)
  line L9581 (135.922, -110.871) -> (135.93, -110.817)
  line L9582 (147.31, -117.21) -> (147.281, -117.219)
  line L9583 (147.34, -117.204) -> (147.31, -117.21)
  line L9584 (127.388, -113.578) -> (127.356, -113.586)
  line L9585 (149.415, -115.136) -> (147.369, -117.182)
  line L9586 (132.284, -122.056) -> (132.185, -122.205)
  line L9587 (127.421, -113.574) -> (127.388, -113.578)
  line L9588 (149.43, -115.109) -> (149.415, -115.136)
  line L9589 (135.941, -110.995) -> (135.922, -110.871)
  line L9590 (124.13, -113.568) -> (124.119, -113.566)
  line L9591 (122.91, -114.1) -> (122.882, -114.118)
  line L9592 (147.929, -102.867) -> (147.902, -102.92)
  line L9593 (147.902, -102.92) -> (149.415, -104.433)
  line L9594 (128.336, -112.631) -> (128.332, -112.664)
  line L9595 (128.302, -112.711) -> (128.284, -112.74)
  line L9596 (132.293, -121.345) -> (132.352, -121.513)
  line L9597 (128.326, -112.674) -> (128.323, -112.685)
  line L9598 (128.284, -112.74) -> (127.497, -113.527)
  line L9599 (128.343, -112.599) -> (128.336, -112.631)
  line L9600 (124.065, -113.527) -> (123.875, -113.338)
  line L9601 (136.087, -111.195) -> (135.998, -111.106)
  line L9602 (132.372, -121.713) -> (132.347, -121.89)
  line L9603 (149.452, -104.521) -> (149.452, -115.048)
  line L9604 (149.448, -115.07) -> (149.449, -115.075)
  line L9605 (127.468, -113.545) -> (127.442, -113.566)
  line L9606 (136.22, -117.219) -> (132.217, -121.222)
  line L9607 (147.345, -117.2) -> (147.34, -117.204)
  line L9608 (132.347, -121.89) -> (132.284, -122.056)
  line L9609 (135.998, -111.106) -> (135.941, -110.995)
  line L9610 (132.372, -121.691) -> (132.372, -121.713)
  line L9611 (147.949, -102.743) -> (147.929, -102.867)
  line L9612 (123.673, -113.338) -> (122.91, -114.1)
  line L9613 (132.352, -121.513) -> (132.372, -121.691)
  line L9614 (149.447, -115.077) -> (149.446, -115.083)
  line L9615 (147.281, -117.219) -> (136.22, -117.219)
  line L9616 (132.217, -121.222) -> (132.293, -121.345)
  line L9617 (149.415, -104.433) -> (149.428, -104.45)
  line L9618 (149.443, -104.491) -> (149.452, -104.521)
  line L9619 (123.875, -113.338) -> (123.774, -113.354)
  line L9620 (124.173, -113.578) -> (124.14, -113.574)
  line L9621 (124.14, -113.574) -> (124.13, -113.568)
  line L9622 (128.734, -110.817) -> (128.343, -111.208)
  line L9623 (130.794, -121.502) -> (130.855, -121.335)
  line L9624 (136.08, -117.006) -> (136.098, -116.992)
  line L9625 (130.952, -121.185) -> (131.079, -121.06)
  line L9626 (136.169, -116.969) -> (147.229, -116.969)
  line L9627 (149.202, -104.573) -> (147.725, -103.096)
  line L9628 (130.855, -121.335) -> (130.952, -121.185)
  line L9629 (131.378, -122.467) -> (131.211, -122.405)
  line L9630 (147.425, -102.363) -> (147.549, -102.343)
  line L9631 (149.844, -102.129) -> (149.863, -102.253)
  line L9632 (149.436, -104.461) -> (149.443, -104.491)
  line L9633 (147.351, -117.196) -> (147.348, -117.199)
  line L9634 (131.755, -120.912) -> (131.923, -120.972)
  line L9635 (131.902, -122.419) -> (131.733, -122.474)
  line L9636 (149.202, -114.996) -> (149.202, -104.573)
  line L9637 (132.056, -122.328) -> (131.902, -122.419)
  line L9638 (147.403, -117.78) -> (147.4, -117.783)
  line L9639 (149.938, -115.238) -> (149.923, -115.265)
  line L9640 (147.549, -103.143) -> (147.425, -103.123)
  line L9641 (147.725, -103.096) -> (147.672, -103.123)
  line L9642 (147.313, -102.419) -> (147.425, -102.363)
  line L9643 (131.4, -120.909) -> (131.578, -120.891)
  line L9644 (147.348, -117.199) -> (147.345, -117.2)
  line L9645 (149.428, -104.45) -> (149.432, -104.453)
  line L9646 (131.578, -120.891) -> (131.755, -120.912)
  line L9647 (147.229, -116.969) -> (149.202, -114.996)
  line L9648 (136.098, -116.992) -> (136.101, -116.989)
  line L9649 (136.139, -116.978) -> (136.169, -116.969)
  line L9650 (147.369, -117.182) -> (147.351, -117.196)
  line L9651 (149.432, -104.453) -> (149.433, -104.456)
  line L9652 (130.938, -122.179) -> (130.846, -122.026)
  line L9653 (131.923, -120.972) -> (132.04, -121.046)
  line L9654 (132.185, -122.205) -> (132.056, -122.328)
  line L9655 (149.452, -115.048) -> (149.448, -115.07)
  line L9656 (130.789, -121.857) -> (130.772, -121.679)
  line L9657 (136.101, -116.989) -> (136.104, -116.988)
  line L9658 (130.772, -121.679) -> (130.794, -121.502)
  line L9659 (136.104, -116.988) -> (136.109, -116.984)
  line L9660 (130.846, -122.026) -> (130.789, -121.857)
  line L9661 (131.231, -120.967) -> (131.4, -120.909)
  line L9662 (131.733, -122.474) -> (131.555, -122.49)
  line L9663 (132.04, -121.046) -> (136.08, -117.006)
  line L9664 (149.787, -102.018) -> (149.844, -102.129)
  line L9665 (136.109, -116.984) -> (136.139, -116.978)
  line L9666 (131.555, -122.49) -> (131.378, -122.467)
  line L9667 (131.062, -122.307) -> (130.938, -122.179)
  line L9668 (131.211, -122.405) -> (131.062, -122.307)
  line L9669 (131.079, -121.06) -> (131.231, -120.967)
  line L9670 (149.923, -115.265) -> (147.421, -117.767)
  line L9671 (133.619, -121.06) -> (133.771, -120.967)
  line L9672 (133.492, -121.185) -> (133.619, -121.06)
  line L9673 (147.425, -103.123) -> (147.313, -103.067)
  line L9674 (134.273, -122.474) -> (134.095, -122.49)
  line L9675 (147.333, -117.803) -> (138.176, -117.803)
  line L9676 (134.833, -121.345) -> (134.892, -121.513)
  line L9677 (149.863, -102.253) -> (149.845, -102.369)
  line L9678 (133.771, -120.967) -> (133.94, -120.909)
  line L9679 (133.94, -120.909) -> (134.118, -120.891)
  line L9680 (134.118, -120.891) -> (134.295, -120.912)
  line L9681 (147.672, -103.123) -> (147.549, -103.143)
  line L9682 (149.94, -102.421) -> (149.96, -102.489)
  line L9683 (149.845, -102.369) -> (149.887, -102.375)
  line L9684 (147.549, -102.343) -> (147.672, -102.363)
  line L9685 (149.957, -115.203) -> (149.955, -115.205)
  line L9686 (134.824, -122.056) -> (134.725, -122.205)
  line L9687 (133.602, -122.307) -> (133.478, -122.179)
  line L9688 (134.442, -122.419) -> (134.273, -122.474)
  line L9689 (149.96, -102.489) -> (149.96, -115.176)
  line L9690 (147.225, -102.978) -> (147.168, -102.867)
  line L9691 (149.96, -115.176) -> (149.956, -115.198)
  line L9692 (133.312, -121.679) -> (133.334, -121.502)
  line L9693 (133.334, -121.502) -> (133.395, -121.335)
  line L9694 (147.4, -117.783) -> (147.398, -117.784)
  line L9695 (147.421, -117.767) -> (147.403, -117.78)
  line L9696 (149.954, -115.212) -> (149.938, -115.238)
  line L9697 (147.168, -102.619) -> (147.225, -102.508)
  line L9698 (149.698, -101.929) -> (149.787, -102.018)
  line L9699 (134.757, -121.222) -> (134.833, -121.345)
  line L9700 (133.918, -122.467) -> (133.751, -122.405)
  line L9701 (138.176, -117.803) -> (134.757, -121.222)
  line L9702 (134.912, -121.713) -> (134.887, -121.89)
  line L9703 (134.887, -121.89) -> (134.824, -122.056)
  line L9704 (133.329, -121.857) -> (133.312, -121.679)
  line L9705 (133.751, -122.405) -> (133.602, -122.307)
  line L9706 (149.955, -115.205) -> (149.954, -115.212)
  line L9707 (147.225, -102.508) -> (147.313, -102.419)
  line L9708 (149.887, -102.375) -> (149.94, -102.421)
  line L9709 (134.892, -121.513) -> (134.912, -121.691)
  line L9710 (147.313, -103.067) -> (147.225, -102.978)
  line L9711 (149.956, -115.198) -> (149.957, -115.203)
  line L9712 (147.168, -102.867) -> (147.149, -102.743)
  line L9713 (147.149, -102.743) -> (147.168, -102.619)
  line L9714 (149.587, -101.873) -> (149.698, -101.929)
  line L9715 (134.596, -122.328) -> (134.442, -122.419)
  line L9716 (133.478, -122.179) -> (133.386, -122.026)
  line L9717 (133.395, -121.335) -> (133.492, -121.185)
  line L9718 (134.725, -122.205) -> (134.596, -122.328)
  line L9719 (150.022, -95.9576) -> (150.022, -97.9276)
  line L9720 (150.022, -97.9276) -> (150.533, -98.4382)
  line L9721 (137.452, -121.691) -> (137.452, -121.713)
  line L9722 (133.386, -122.026) -> (133.329, -121.857)
  line L9723 (138.095, -117.562) -> (138.124, -117.553)
  line L9724 (134.58, -121.046) -> (138.036, -117.59)
  line L9725 (150.048, -95.1926) -> (150.16, -95.2494)
  line L9726 (134.095, -122.49) -> (133.918, -122.467)
  line L9727 (149.587, -102.633) -> (149.463, -102.653)
  line L9728 (134.463, -120.972) -> (134.58, -121.046)
  line L9729 (150.16, -95.2494) -> (150.248, -95.3379)
  line L9730 (149.083, -102.129) -> (149.14, -102.018)
  line L9731 (147.591, -118.342) -> (147.588, -118.343)
  line L9732 (150.561, -98.4971) -> (150.569, -98.5266)
  line L9733 (147.398, -117.784) -> (147.392, -117.788)
  line L9734 (134.912, -121.691) -> (134.912, -121.713)
  line L9735 (138.054, -117.576) -> (138.057, -117.573)
  line L9736 (138.036, -117.59) -> (138.054, -117.576)
  line L9737 (149.228, -101.929) -> (149.34, -101.873)
  line L9738 (150.305, -95.6966) -> (150.248, -95.8081)
  line L9739 (149.463, -101.853) -> (149.587, -101.873)
  line L9740 (150.248, -95.3379) -> (150.305, -95.4494)
  line L9741 (138.057, -117.573) -> (138.06, -117.572)
  line L9742 (149.063, -102.253) -> (149.083, -102.129)
  line L9743 (147.392, -117.788) -> (147.362, -117.795)
  line L9744 (149.228, -102.577) -> (149.14, -102.488)
  line L9745 (147.281, -117.553) -> (149.71, -115.125)
  line L9746 (150.564, -115.352) -> (150.547, -115.377)
  line L9747 (150.533, -98.4382) -> (150.546, -98.456)
  line L9748 (149.71, -115.125) -> (149.71, -102.565)
  line L9749 (149.463, -102.653) -> (149.34, -102.633)
  line L9750 (149.34, -101.873) -> (149.463, -101.853)
  line L9751 (137.432, -121.513) -> (137.452, -121.691)
  line L9752 (150.569, -115.316) -> (150.566, -115.338)
  line L9753 (138.06, -117.572) -> (138.065, -117.568)
  line L9754 (150.325, -95.573) -> (150.305, -95.6966)
  line L9755 (138.124, -117.553) -> (147.281, -117.553)
  line L9756 (134.295, -120.912) -> (134.463, -120.972)
  line L9757 (138.065, -117.568) -> (138.095, -117.562)
  line L9758 (149.14, -102.018) -> (149.228, -101.929)
  line L9759 (147.362, -117.795) -> (147.333, -117.803)
  line L9760 (149.71, -102.565) -> (149.698, -102.577)
  line L9761 (150.248, -95.8081) -> (150.16, -95.8966)
  line L9762 (149.698, -102.577) -> (149.587, -102.633)
  line L9763 (149.14, -102.488) -> (149.083, -102.377)
  line L9764 (149.34, -102.633) -> (149.228, -102.577)
  line L9765 (149.083, -102.377) -> (149.063, -102.253)
  line L9766 (150.305, -95.4494) -> (150.325, -95.573)
  line L9767 (136.835, -120.912) -> (137.003, -120.972)
  line L9768 (140.076, -118.121) -> (140.106, -118.112)
  line L9769 (136.018, -122.179) -> (135.926, -122.026)
  line L9770 (137.427, -121.89) -> (137.364, -122.056)
  line L9771 (136.291, -122.405) -> (136.142, -122.307)
  line L9772 (147.583, -118.347) -> (147.553, -118.353)
  line L9773 (150.566, -115.343) -> (150.565, -115.345)
  line L9774 (150.565, -115.345) -> (150.564, -115.352)
  line L9775 (135.926, -122.026) -> (135.869, -121.857)
  line L9776 (136.982, -122.419) -> (136.813, -122.474)
  line L9777 (136.311, -120.967) -> (136.48, -120.909)
  line L9778 (135.935, -121.335) -> (136.032, -121.185)
  line L9779 (140.106, -118.112) -> (147.471, -118.112)
  line L9780 (137.12, -121.046) -> (140.017, -118.149)
  line L9781 (150.55, -98.4618) -> (150.554, -98.467)
  line L9782 (150.554, -98.467) -> (150.561, -98.4971)
  line L9783 (137.364, -122.056) -> (137.265, -122.205)
  line L9784 (136.658, -120.891) -> (136.835, -120.912)
  line L9785 (150.16, -95.8966) -> (150.048, -95.9535)
  line L9786 (136.458, -122.467) -> (136.291, -122.405)
  line L9787 (137.136, -122.328) -> (136.982, -122.419)
  line L9788 (136.159, -121.06) -> (136.311, -120.967)
  line L9789 (150.569, -98.5266) -> (150.569, -115.316)
  line L9790 (147.523, -118.362) -> (140.157, -118.362)
  line L9791 (150.048, -95.9535) -> (150.022, -95.9576)
  line L9792 (150.546, -98.456) -> (150.549, -98.4591)
  line L9793 (137.297, -121.222) -> (137.373, -121.345)
  line L9794 (135.869, -121.857) -> (135.852, -121.679)
  line L9795 (136.032, -121.185) -> (136.159, -121.06)
  line L9796 (136.48, -120.909) -> (136.658, -120.891)
  line L9797 (140.038, -118.132) -> (140.041, -118.131)
  line L9798 (135.852, -121.679) -> (135.874, -121.502)
  line L9799 (140.041, -118.131) -> (140.046, -118.127)
  line L9800 (150.566, -115.338) -> (150.566, -115.343)
  line L9801 (147.594, -118.339) -> (147.591, -118.342)
  line L9802 (147.612, -118.325) -> (147.594, -118.339)
  line L9803 (136.635, -122.49) -> (136.458, -122.467)
  line L9804 (137.003, -120.972) -> (137.12, -121.046)
  line L9805 (135.874, -121.502) -> (135.935, -121.335)
  line L9806 (150.547, -115.377) -> (150.533, -115.404)
  line L9807 (150.549, -98.4591) -> (150.55, -98.4618)
  line L9808 (150.319, -115.264) -> (150.319, -98.5784)
  line L9809 (137.452, -121.713) -> (137.427, -121.89)
  line L9810 (150.533, -115.404) -> (147.612, -118.325)
  line L9811 (137.373, -121.345) -> (137.432, -121.513)
  line L9812 (147.553, -118.353) -> (147.523, -118.362)
  line L9813 (147.588, -118.343) -> (147.583, -118.347)
  line L9814 (140.157, -118.362) -> (137.297, -121.222)
  line L9815 (139.837, -121.222) -> (139.913, -121.345)
  line L9816 (149.795, -98.05) -> (149.792, -98.0469)
  line L9817 (139.972, -121.513) -> (139.992, -121.691)
  line L9818 (151.277, -115.49) -> (151.278, -115.495)
  line L9819 (151.259, -115.53) -> (151.244, -115.557)
  line L9820 (149.601, -95.8081) -> (149.544, -95.6966)
  line L9821 (149.772, -95.9387) -> (149.772, -95.9386)
  line L9822 (151.257, -97.821) -> (151.261, -97.8241)
  line L9823 (151.002, -97.2346) -> (151.022, -97.3582)
  line L9824 (136.813, -122.474) -> (136.635, -122.49)
  line L9825 (149.544, -95.4494) -> (149.601, -95.3379)
  line L9826 (142.062, -118.997) -> (139.837, -121.222)
  line L9827 (150.746, -96.9778) -> (150.857, -97.0346)
  line L9828 (136.142, -122.307) -> (136.018, -122.179)
  line L9829 (150.975, -97.5348) -> (151.244, -97.8032)
  line L9830 (149.791, -98.0442) -> (149.787, -98.039)
  line L9831 (151.261, -97.8241) -> (151.261, -97.8268)
  line L9832 (149.809, -98.0678) -> (149.795, -98.05)
  line L9833 (150.857, -97.0346) -> (150.946, -97.1231)
  line L9834 (151.244, -97.8032) -> (151.257, -97.821)
  line L9835 (140.046, -118.127) -> (140.076, -118.121)
  line L9836 (150.946, -97.1231) -> (151.002, -97.2346)
  line L9837 (149.925, -95.173) -> (150.048, -95.1926)
  line L9838 (149.601, -95.3379) -> (149.69, -95.2494)